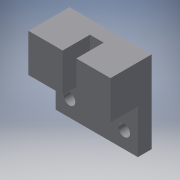
# Autodesk Inventor part: XCartBeltClamp
Saved by Autodesk Inventor 2019 (Build 230136000, 136)
## iProperties
Created: 2019-08-21
Part Number: XCartBeltClamp
Material: Generic
Document SubType Name: Modeling
Designer: Bruno
Density: 1 g/cm^3
Appearance: Default
Author: Bruno
Autodesk Inventor part; units mm, degrees
ref_plane "YZ Plane" through (0, 0, 0) normal (1, 0, 0) x (0, 1, 0)
ref_plane "XZ Plane" through (0, 0, 0) normal (0, 1, 0) x (-1, 0, 0)
ref_plane "XY Plane" through (0, 0, 0) normal (0, 0, 1) x (1, 0, 0)
sketch "Sketch1" plane through (0, 0, 0) normal (0, 0, 1) x (1, 0, 0)
  line L0 (17.8338, 5.1078) -> (-12.1662, 5.1078)
  line L1 (-12.1662, 5.1078) -> (-12.1662, 35.1078)
  line L2 (-12.1662, 35.1078) -> (17.8338, 35.1078)
  line L3 (17.8338, 35.1078) -> (17.8338, 5.1078)
  circle A0 centre (12.8338, 11.1078) radius 2.125
  circle A1 centre (-7.1662, 11.1078) radius 2.125
  line L4 (12.8338, 11.1078) -> (17.8338, 11.1078) construction
  line L5 (-7.1662, 11.1078) -> (-12.1662, 11.1078) construction
  line L6 (12.8338, 11.1078) -> (12.8338, 5.1078) construction
  dimension "d2" = 30
  dimension "d3" = 30
  dimension "d10" = 4.25
  dimension "d11" = 4.25
  dimension "d12" = 5
  dimension "d13" = 6
  constraints: 14 end point, 4 perpendicular, 3 point on line, 2 centre point, 2 collinear, 2 horizontal, 2 parallel, 1 vertical
  measures "d2" distance of L0.end L1.end
  measures "d3" distance of L1.end L2.end
  measures "d10" diameter of A0
  measures "d11" diameter of A1
  measures "d12" distance of L5.start L5.end
  measures "d13" distance of L4.start L6.end
extrude "Extrusion1" add sketch "Sketch1" along normal blind 5
sketch "Sketch2" plane through (0, 0, 5) normal (0, 0, 1) x (1, 0, 0)
  line L0 (-12.1662, 35.1078) -> (-12.1662, 5.1078) projected
  line L1 (-12.1662, 21.1078) -> (0.3338, 21.1078)
  line L2 (0.3338, 21.1078) -> (0.3338, 35.1078)
  line L3 (17.8338, 35.1078) -> (-12.1662, 35.1078) projected
  line L4 (0.3338, 35.1078) -> (-12.1662, 35.1078)
  line L5 (-12.1662, 35.1078) -> (-12.1662, 21.1078)
  line L6 (17.8338, 5.1078) -> (17.8338, 35.1078) projected
  line L7 (17.8338, 21.1078) -> (5.3338, 21.1078)
  line L8 (5.3338, 21.1078) -> (5.3338, 35.1078)
  line L9 (17.8338, 35.1078) -> (17.8338, 21.1078)
  point P0 (0, 0)
  dimension "d6" = 5
  dimension "d7" = 14
  constraints: 14 end point, 3 point on line, 2 collinear, 2 equal length, 2 horizontal, 2 perpendicular, 1 parallel
  measures "d6" distance between parallel lines of L8 L2
  measures "d7" distance of L7.end L8.end
extrude "Extrusion2" add sketch "Sketch2" along normal blind 10
body "Solid1"
